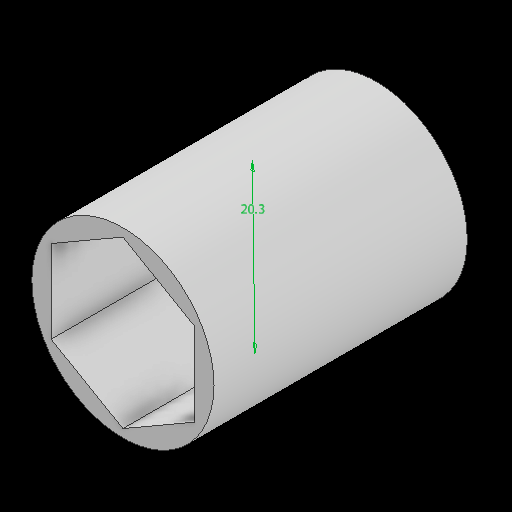
# Autodesk Inventor part: RodMotorMount
Saved by Autodesk Inventor 2025 (Build 290162000, 162)
## iProperties
Created: 2024-11-18
Part Number: RodMotorMount
Material: Generic
Document SubType Name: Modeling
Designer: Trevor
Density: 1 g/cm^3
Appearance: Default
Author: Trevor
Autodesk Inventor part; units mm, degrees
ref_plane "YZ Plane" through (0, 0, 0) normal (1, 0, 0) x (0, 1, 0)
ref_plane "XZ Plane" through (0, 0, 0) normal (0, 1, 0) x (-1, 0, 0)
sketch "Sketch1" plane through (0, 0, 0) normal (0, 0, 1) x (1, 0, 0)
  line L0 (-2.4408, -0.5408) -> (-1.2026, 2.1918) projected
  arc A0 (-2.4408, -0.5408) -> (-1.2026, 2.1918) centre (0, 0) ccw projected
  circle A1 centre (0, 0) radius 3.5
  line L1 (-3.6608, -0.2297) -> (-3.4925, -0.2297)
  line L2 (-3.4925, 0.2297) -> (-3.6608, 0.2297)
  line L3 (-3.6608, 0.2297) -> (-3.6608, -0.2297)
  line L4 (-3.6608, -0.2297) -> (-3.5, 0) construction
  line L5 (-3.5, 0) -> (-3.6608, 0.2297) construction
  point P0 (0, 0)
  dimension "d0" = 7
  constraints: 10 end point, 3 point on circle, 1 centre point, 1 coincident, 1 horizontal, 1 parallel
  measures "d0" diameter of A1
ref_plane "Work Plane1" through (-2, -2, 15) normal (0, 0, 1) x (1, 0, 0)
extrude "Extrusion1" add sketch "Sketch1" along normal up to surface (15 mm away) contours A1
sketch "Sketch2" plane through (0, 0, 15) normal (0, 0, 1) x (1, 0, 0)
  arc A0 (-2.4408, -0.5408) -> (-1.2026, 2.1918) centre (0, 0) ccw projected
  line L0 (-1.2026, 2.1918) -> (-2.4408, -0.5408) projected
  circle A1 centre (0, 0) radius 3.5 projected
  arc A2 (-2.702, -0.5115) -> (-1.3968, 2.3688) centre (0, 0) ccw
  line L1 (-2.702, -0.5115) -> (-1.3968, 2.3688)
  point P0 (0, 0)
  dimension "d9" = 0.25
  constraints: 2 end point, 2 point on circle, 1 centre point, 1 other
  measures "d9" radial gap between concentric circles of A0 A2
extrude "Extrusion2" cut sketch "Sketch2" against normal up to surface (15 mm away) contours L1 A2
sketch "Sketch6" plane through (0, 0, 15) normal (0, 0, 1) x (1, 0, 0)
  circle A0 centre (0, 0) radius 10.15
  line L0 (0, 10.15) -> (8.7902, 5.075)
  line L1 (8.7902, 5.075) -> (8.7902, -5.075)
  line L2 (8.7902, -5.075) -> (0, -10.15)
  line L3 (0, -10.15) -> (-8.7902, -5.075)
  line L4 (-8.7902, -5.075) -> (-8.7902, 5.075)
  line L5 (-8.7902, 5.075) -> (0, 10.15)
  arc A1 (-2.702, -0.5115) -> (-1.3968, 2.3688) centre (0, 0) ccw projected
  line L6 (-1.3968, 2.3688) -> (-2.702, -0.5115) projected
  circle A2 centre (0, 0) radius 3.5 projected
  point P0 (0, -10.15)
  point P1 (0, -10.15)
  dimension "d20" = 20.3
  constraints: 12 end point, 2 coincident, 16 other
extrude "Extrusion5" add sketch "Sketch6" along normal blind 8 contours A0 L1 | L0 A0 | A0 L2 | L5 A0 | A0 L3 | L4 A0
extrude "Extrusion6" add sketch "Sketch6" against normal up to surface (15 mm away) contours A0 L1 | L0 A0 | L1 L2 L3 L4 L5 L0 | A0 L2 | L5 A0 | A0 L3 | L4 A0
sketch "Sketch7" plane through (0, 0, 0) normal (0, 0, -1) x (-1, 0, 0)
  circle A0 centre (0, 0) radius 10.15 projected
  arc A1 (1.3968, 2.3688) -> (2.702, -0.5115) centre (0, 0) ccw projected
  line L0 (1.3968, 2.3688) -> (2.702, -0.5115) projected
  circle A2 centre (0, 0) radius 11.15
  dimension "d25" = 1
  constraints: 1 centre point
  measures "d25" radial gap between concentric circles of A0 A2
extrude "Extrusion7" add sketch "Sketch7" against normal up to surface (23 mm away) contours A2
sketch "Sketch8" plane through (0, 0, 23) normal (0, 0, 1) x (1, 0, 0)
  circle A0 centre (0, 0) radius 11.15 projected
  line L0 (-8.7902, -5.075) -> (-8.7902, 5.075) projected
  line L1 (-8.7902, 5.075) -> (0, 10.15) projected
  line L2 (0, 10.15) -> (8.7902, 5.075) projected
  line L3 (8.7902, 5.075) -> (8.7902, -5.075) projected
  line L4 (8.7902, -5.075) -> (0, -10.15) projected
  line L5 (0, -10.15) -> (-8.7902, -5.075) projected
  point P0 (0, 0)
extrude "Extrusion8" add sketch "Sketch8" along normal blind 8
body "Solid1"
